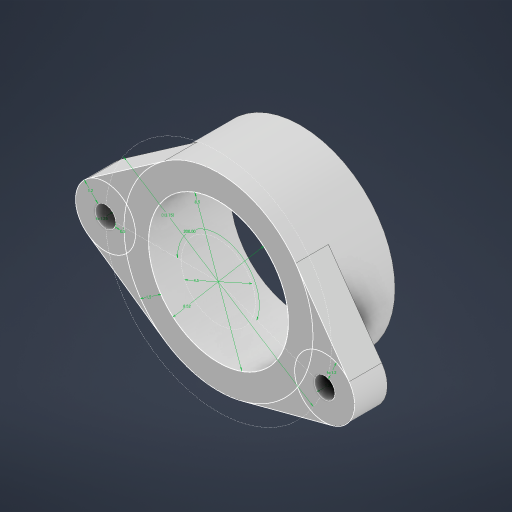
# Autodesk Inventor part: motorauxiliary
Saved by Autodesk Inventor 2023.5 (Build 275446000, 446)
## iProperties
Created: 2024-12-07
Part Number: motorauxiliary
Material: 一般
Document SubType Name: Modeling
Designer: IshiiLabHonda
Density: 1 g/cm^3
Appearance: 既定
Author: IshiiLabHonda
Autodesk Inventor part; units mm, degrees
ref_plane "YZ Plane" through (0, 0, 0) normal (1, 0, 0) x (0, 1, 0)
ref_plane "XZ Plane" through (0, 0, 0) normal (0, 1, 0) x (-1, 0, 0)
ref_plane "XY Plane" through (0, 0, 0) normal (0, 0, 1) x (1, 0, 0)
sketch "スケッチ1" plane through (0, 0, 0) normal (0, 0, 1) x (1, 0, 0)
  circle A0 centre (0, 0) radius 2.25 construction
  circle A1 centre (0, 0) radius 4.26
  circle A2 centre (0, 0) radius 5.75
  circle A3 centre (-6.875, 0) radius 0.625
  circle A4 centre (6.4604, -2.3514) radius 0.625
  circle A5 centre (0, 0) radius 6.875 construction
  circle A6 centre (-6.875, 0) radius 1.825
  circle A7 centre (6.4604, -2.3514) radius 1.825
  line L0 (-7.9169, 1.4983) -> (-3.2827, 4.7208)
  line L1 (-7.9169, -1.4983) -> (-3.2827, -4.7208)
  line L2 (6.927, -4.1157) -> (1.4701, -5.5589)
  line L3 (4.6994, 3.3134) -> (7.9519, -1.2998)
  line L4 (6.4604, -2.3514) -> (0, 0) construction
  line L5 (0, 0) -> (-6.875, 0) construction
  circle A8 centre (0, 0) radius 4.25
  point P0 (5.7086, -0.6884)
  point P1 (4.8156, -3.1421)
  point P2 (-5.5998, 1.3056)
  point P3 (-5.5998, -1.3056)
  dimension "d2" = 4.5
  dimension "d3" = 8.52
  dimension "d5" = 1.25
  dimension "d6" = 1.25
  dimension "d7" = 1.2
  dimension "d8" = 1.2
  dimension "d9" = 0.5
  dimension "d18" = 200
  dimension "d22" = 13.75
  dimension "d23" = 8.5
  dimension "d24" = 1.5
  constraints: 12 end point, 10 point on circle, 9 centre point, 8 coincident, 8 tangent, 1 horizontal
  measures "d2" diameter of A0
  measures "d3" diameter of A1
  measures "d5" diameter of A4
  measures "d6" diameter of A3
  measures "d7" radial gap between concentric circles of A6 A3
  measures "d8" radial gap between concentric circles of A7 A4
  measures "d22" diameter of A5
  measures "d23" diameter of A8
  measures "d24" radial gap between concentric circles of A2 A8
extrude "押し出し1" add sketch "スケッチ1" against normal blind 5 contours A2 A7 A6 | A2 A7 | A6 A2 picked at (5.2008, -1.8194) picked at (-5.5055, 0)
extrude "押し出し3" add sketch "スケッチ1" against normal blind 2 contours A2 A6 L0 | A2 A6 | A2 L1 A6 picked at (-5.951, -0.7528)
extrude "押し出し4" add sketch "スケッチ1" against normal blind 2 contours A2 L3 A7 | A7 A2 | A7 L2 A2 picked at (5.8283, -1.3347)
equation "\"d6\" = d5"
equation "\"d8\" = d7"
